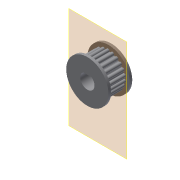
# Autodesk Inventor part: 30_CUBE_openXY_gear_2mmbelt_NEMA
Saved by Autodesk Inventor 2019 (Build 230136000, 136)
## iProperties
Created: 2020-03-17
Part Number: 30_CUBE_openXY_gear_2mmbelt_NEMA
Material: Generic
Document SubType Name: Modeling
Designer: diederichbenedict
Density: 1 g/cm^3
Appearance: Default
Author: diederichbenedict
Autodesk Inventor part; units mm, degrees
ref_plane "YZ Plane" through (0, 0, 0) normal (1, 0, 0) x (0, 1, 0)
ref_plane "XZ Plane" through (0, 0, 0) normal (0, 1, 0) x (-1, 0, 0)
ref_plane "XY Plane" through (0, 0, 0) normal (0, 0, 1) x (1, 0, 0)
ref_plane "Work Plane1" through (0, 0, 0) normal (0, 0, 1) x (1, 0, 0)
sketch "Sketch1" plane through (0, 0, 0) normal (0, 0, 1) x (1, 0, 0)
  circle A0 centre (4.149, 7.0628) radius 1.6 projected
  circle A1 centre (4.149, 7.0628) radius 1.6 construction
  line L0 (4.149, 7.0628) -> (4.1493, 3.0628) construction
  arc A2 (3.1573, 3.0949) -> (3.2673, 3.069) centre (4.149, 7.0628) ccw
  arc A3 (3.1377, 3.0998) -> (3.2673, 3.069) centre (4.149, 7.0628) ccw
  arc A4 (5.599, 10.8872) -> (5.3687, 10.9668) centre (4.149, 7.0628) ccw
  arc A5 (7.0291, 9.9668) -> (6.8511, 10.1332) centre (4.149, 7.0628) ccw
  arc A6 (7.0291, 9.9668) -> (6.8511, 10.1332) centre (4.149, 7.0628) ccw
  arc A7 (5.599, 10.8872) -> (5.7734, 10.9392) centre (5.6521, 11.0275) ccw construction
  arc A8 (6.8154, 10.3117) -> (6.8511, 10.1332) centre (6.9502, 10.2458) ccw construction
  arc A9 (5.599, 10.8872) -> (5.7734, 10.9392) centre (5.6521, 11.0275) ccw
  arc A10 (6.8154, 10.3117) -> (6.8511, 10.1332) centre (6.9502, 10.2458) ccw
  arc A11 (6.8154, 10.3117) -> (5.7734, 10.9392) centre (6.3283, 10.6818) ccw
  arc A12 (5.599, 10.8872) -> (6.8511, 10.1332) centre (4.149, 7.0628) ccw
  arc A13 (2.649, 9.0628) -> (5.649, 9.0628) centre (4.149, 7.0628) ccw construction
  line L1 (5.649, 9.0628) -> (2.649, 9.0628) construction
  arc A14 (2.5838, 9.2628) -> (5.7143, 9.2628) centre (4.149, 7.0628) ccw
  line L2 (2.5838, 9.2628) -> (5.7143, 9.2628)
  arc A15 (6.5952, 12.5415) -> (7.8473, 11.7875) centre (4.149, 7.0628) ccw
  line L3 (4.149, 7.0628) -> (6.3283, 10.6818) construction
  line L4 (6.2911, 10.6199) -> (7.2443, 12.2028) construction
  line L5 (5.599, 10.8872) -> (6.5952, 12.5415) construction
  line L6 (6.8511, 10.1332) -> (7.8473, 11.7875) construction
  circle A16 centre (4.149, 7.0628) radius 4.09 construction
  line L7 (7.2443, 12.2028) -> (7.5355, 12.6864) construction
  arc A17 (7.9208, 11.9095) -> (6.6402, 12.6096) centre (7.3001, 12.2955) ccw construction
  circle A18 centre (4.149, 7.0628) radius 6.1213 construction
  line L8 (6.8154, 10.3117) -> (8.0693, 12.3939) construction
  line L9 (5.7734, 10.9392) -> (6.853, 12.732) construction
  arc A19 (7.8123, 11.967) -> (6.7702, 12.5945) centre (7.3001, 12.2955) ccw
  circle A20 centre (4.149, 7.0628) radius 6
  arc A21 (7.8473, 11.7875) -> (6.5796, 12.5485) centre (4.137, 7.0428) ccw
  arc A22 (6.5952, 12.5415) -> (6.7702, 12.5945) centre (6.6453, 12.6917) ccw
  arc A23 (7.8123, 11.967) -> (7.8473, 11.7875) centre (7.9336, 11.8975) ccw
  point P0 (0, 0)
  point P1 (7.0406, 11.0098)
  dimension "d0" = 3.2
  dimension "d15" = 0.2
  dimension "d19" = 12
  dimension "d20" = 0.6117
  constraints: 41 point on circle, 22 centre point, 18 end point, 8 coincident, 4 concentric, 4 parallel, 3 point on line, 2 collinear, 15 other
  measures "d0" diameter of A1
  measures "d15" radial gap between concentric circles of A13 A14
  measures "d19" diameter of A15
  measures "d20" radius of A11
extrude "Extrusion1" add sketch "Sketch1" along normal blind 7 contours A3 A12 A4 A9 A11 A10 A5 A2 | A20 A15 | A22 A19 A23 A20
pattern_circular "Circular Pattern1" count 22 over 360 about axis through (4.149, 7.0628, 0) along (0, 0, 1) of "Extrusion1"
sketch "Sketch2" plane through (0, 0, 0) normal (0, 0, -1) x (-1, 0, 0)
  circle A0 centre (-4.149, 7.0628) radius 1.6 projected
  circle A1 centre (-4.149, 7.0628) radius 8
  point P0 (0, 0)
  dimension "d10" = 16
  constraints: 1 centre point, 1 coincident
  measures "d10" diameter of A1
extrude "Extrusion2" add sketch "Sketch2" along normal blind 1
sketch "Sketch3" plane through (0, 0, 7) normal (0, 0, 1) x (1, 0, 0)
  circle A0 centre (4.149, 7.0628) radius 1.6 projected
  circle A1 centre (4.149, 7.0628) radius 8 projected
  point P0 (0, 0)
extrude "Extrusion3" add sketch "Sketch3" along normal blind 1
sketch "Sketch4" plane through (4.149, 7.0628, 8) normal (0, 0, 1) x (1, 0, 0)
  arc A0 (-1.5, 2) -> (1.5, 2) centre (0, 0) ccw projected
  line L0 (1.5, 2) -> (-1.5, 2) projected
  arc A1 (-1.5652, 2.2) -> (1.5652, 2.2) centre (0, 0) ccw
  line L1 (-1.5652, 2.2) -> (1.5652, 2.2)
  point P0 (-4.149, -7.0628)
  dimension "d16" = 0.2
  constraints: 2 end point, 2 point on circle, 1 centre point, 1 other
  measures "d16" radial gap between concentric circles of A0 A1
extrude "Extrusion4" cut sketch "Sketch4" against normal blind 10 contours L0 A0 | L1 A1
body "Solid1"
